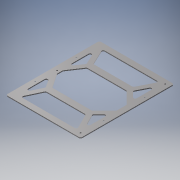
# Autodesk Inventor part: ZBedPlate
Saved by Autodesk Inventor 2016 (Build 200138000, 138)
## iProperties
Category: Sheet Metal
Created: 2015-01-11
Part Number: ZBedPlate
Material: Steel, Alloy
Document SubType Name: Modeling
Designer: Jack
Density: 7.73 g/cm^3
Appearance: Semi-Polished
Mass: 734.813 g
Surface Area: 727.52 cm^2
Volume: 95.0599 cm^3
Author: Jack
Title: Bed Support Plate
Autodesk Inventor part; units mm, degrees
ref_plane "YZ Plane" through (0, 0, 0) normal (1, 0, 0) x (0, 1, 0)
ref_plane "XZ Plane" through (0, 0, 0) normal (0, 1, 0) x (-1, 0, 0)
ref_plane "XY Plane" through (0, 0, 0) normal (0, 0, 1) x (1, 0, 0)
sketch "Sketch1" plane through (0, 0, 0) normal (0, 0, 1) x (1, 0, 0)
  line L0 (0, 0) -> (236.5, 0)
  line L1 (236.5, 0) -> (236.5, 296)
  line L2 (236.5, 296) -> (0, 296)
  line L3 (0, 296) -> (0, 0)
  dimension "d0" = 236.5
  dimension "d1" = 296
  constraints: 8 end point, 2 parallel, 1 horizontal, 1 perpendicular
  measures "d0" distance of L0.start L0.end
  measures "d1" distance of L2.end L0.start
extrude "Extrusion1" add sketch "Sketch1" along normal blind 3
sketch "Sketch2" plane through (0, 0, 3) normal (0, 0, 1) x (1, 0, 0)
  line L0 (0, 0) -> (236.5, 0) projected
  line L1 (236.5, 0) -> (236.5, 296) projected
  line L2 (236.5, 296) -> (0, 296) projected
  line L3 (0, 296) -> (0, 0) projected
  line L4 (207.5752, 278) -> (27.5752, 278)
  line L5 (27.5752, 278) -> (53.2221, 223)
  line L6 (53.2221, 223) -> (179.8118, 223)
  line L7 (179.8118, 223) -> (207.5752, 278)
  line L8 (216.5, 264.6127) -> (190.1661, 212.4446)
  line L9 (190.1661, 212.4446) -> (216.5, 186.1108)
  line L10 (218.5, 164.3118) -> (179.8118, 203)
  line L11 (216.5, 264.6127) -> (216.5, 186.1108)
  line L12 (179.8118, 203) -> (53.2221, 203)
  line L13 (53.2221, 203) -> (22.7929, 157.529)
  line L14 (18, 265.4073) -> (42.6969, 212.4446)
  line L15 (42.6969, 212.4446) -> (18, 175.5396)
  line L16 (18, 175.5396) -> (18, 265.4073)
  line L17 (22.7929, 138.471) -> (53.2221, 93)
  line L18 (53.2221, 93) -> (179.8118, 93)
  line L19 (179.8118, 93) -> (218.5, 131.6882)
  line L20 (218.5, 131.6882) -> (218.5, 164.3118)
  line L21 (216.5, 109.8892) -> (190.1661, 83.5554)
  line L22 (190.1661, 83.5554) -> (216.5, 31.3873)
  line L23 (216.5, 31.3873) -> (216.5, 109.8892)
  line L24 (18, 120.4604) -> (42.6969, 83.5554)
  line L25 (42.6969, 83.5554) -> (18, 30.5927)
  line L26 (18, 30.5927) -> (18, 120.4604)
  line L27 (27.5752, 18) -> (207.5752, 18)
  line L28 (207.5752, 18) -> (179.8118, 73)
  line L29 (179.8118, 73) -> (53.2221, 73)
  line L30 (53.2221, 73) -> (27.5752, 18)
  line L31 (22.7929, 138.471) -> (22.7929, 157.529)
  dimension "d19" = 65
  dimension "d29" = 110
  dimension "d31" = 20
  dimension "d32" = 18
  dimension "d33" = 18
  dimension "d34" = 20
  dimension "d35" = 18
  dimension "d40" = 14
  dimension "d41" = 14
  dimension "d52" = 180
  dimension "d55" = 135
  dimension "d59" = 20
  dimension "d60" = 14
  dimension "d61" = 14
  dimension "d62" = 14
  dimension "d63" = 14
  dimension "d64" = 18
  constraints: 56 end point, 11 parallel, 9 vertical alignment, 8 equal length, 5 vertical, 4 horizontal, 2 horizontal alignment
  measures "d19" angle of L27 L30
  measures "d29" distance between parallel lines of L18 L12
  measures "d31" distance between parallel lines of L6 L12
  measures "d32" distance between parallel lines of L2 L4
  measures "d33" distance between parallel lines of L0 L27
  measures "d34" distance between parallel lines of L1 L11
  measures "d35" distance between parallel lines of L3 L16
  measures "d40" distance between parallel lines of L13 L15
  measures "d41" distance between parallel lines of L9 L10
  measures "d52" distance of L27.start L27.end
  measures "d55" angle of L12 L10
  measures "d59" distance between parallel lines of L29 L18
  measures "d60" distance between parallel lines of L30 L25
  measures "d61" distance between parallel lines of L22 L28
  measures "d62" distance between parallel lines of L8 L7
  measures "d63" distance between parallel lines of L14 L5
  measures "d64" distance between parallel lines of L1 L20
extrude "Extrusion2" cut sketch "Sketch2" against normal up to next contours L7 L6 L5 L4 | L11 L9 L8 | L20 L19 L18 L17 L31 L13 L12 L10 | L14 L15 L16 | L23 L22 L21 | L24 L25 L26 | L30 L29 L28 L27
sketch "Sketch3" plane through (0, 0, 3) normal (0, 0, 1) x (1, 0, 0)
  line L0 (0, 0) -> (236.5, 0) projected
  line L1 (236.5, 0) -> (236.5, 296) projected
  line L2 (236.5, 296) -> (0, 296) projected
  line L3 (0, 296) -> (0, 0) projected
  circle A0 centre (222.5, 282) radius 2.25
  circle A1 centre (14, 148) radius 2.25
  circle A2 centre (222.5, 14) radius 2.25
  dimension "d44" = 4.5
  dimension "d45" = 14
  dimension "d46" = 14
  dimension "d47" = 14
  dimension "d56" = 148
  dimension "d57" = 14
  constraints: 3 centre point, 2 equal radius, 1 vertical alignment
  measures "d44" diameter of A0
  measures "d45" distance from line of L1 A0.centre
  measures "d46" distance from line of L2 A0.centre
  measures "d47" distance from line of L0 A2.centre
  measures "d56" distance from line of L2 A1.centre
  measures "d57" distance from line of L3 A1.centre
extrude "Extrusion3" cut sketch "Sketch3" against normal up to next contours A0 | A1 | A2
fillet "Fillet1" radius 4.7625 28 edges at (27.5752, 18, 1.5) (207.5752, 18, 1.5) (179.8118, 73, 1.5) (53.2221, 73, 1.5) (18, 30.5927, 1.5) (42.6969, 83.5554, 1.5) (18, 120.4604, 1.5) (42.6969, 212.4446, 1.5) (18, 175.5396, 1.5) (18, 265.4073, 1.5) (27.5752, 278, 1.5) (53.2221, 223, 1.5) (179.8118, 223, 1.5) (207.5752, 278, 1.5) (190.1661, 83.5554, 1.5) (216.5, 31.3873, 1.5) (216.5, 109.8892, 1.5) (216.5, 186.1108, 1.5) (190.1661, 212.4446, 1.5) (216.5, 264.6127, 1.5) (218.5, 131.6882, 1.5) (218.5, 164.3118, 1.5) (179.8118, 93, 1.5) (179.8118, 203, 1.5) (53.2221, 203, 1.5) (22.7929, 157.529, 1.5) (22.7929, 138.471, 1.5) (53.2221, 93, 1.5)
fillet "Fillet2" radius 5 4 edges at (236.5, 0, 1.5) (0, 0, 1.5) (0, 296, 1.5) (236.5, 296, 1.5)
sketch "Sketch4" plane through (0, 0, 0) normal (0, 0, -1) x (-1, 0, 0)
  line L0 (-177.8391, 203) -> (-55.7656, 203) projected
  line L1 (-55.7656, 93) -> (-177.8391, 93) projected
  line L2 (-236.5, 5) -> (-236.5, 291) projected
  line L3 (0, 291) -> (0, 5) projected
  point P0 (0, 0)
  point P1 (-10, 213)
  point P2 (-226.5, 213)
  point P3 (-10, 83)
  point P4 (-226.5, 83)
  dimension "d65" = 10
  dimension "d66" = 10
  dimension "d67" = 10
  dimension "d68" = 10
  constraints: 2 horizontal alignment, 2 vertical alignment
  measures "d65" distance from line of point (-10, 213) L0
  measures "d66" distance from line of point (-10, 83) L1
  measures "d67" distance from line of L2 point (-226.5, 83)
  measures "d68" distance from line of L3 point (-10, 83)
hole "Hole1" at (10, 213, 0) at (226.5, 213, 0) at (10, 83, 0) at (226.5, 83, 0) direction (0, 0, 1) diameter 4 end through all countersink diameter 8 countersink angle 90
body "Solid1"
